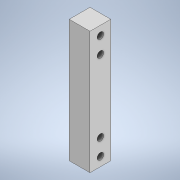
# Autodesk Inventor part: Load_Cell
Saved by Autodesk Inventor 2022 (Build 260153000, 153)
## iProperties
Created: 2022-09-14
Part Number: Load_Cell
Material: Generic
Document SubType Name: Modeling
Designer: tecssupport
Density: 1 g/cm^3
Appearance: Default
Author: tecssupport
Autodesk Inventor part; units mm, degrees
ref_plane "YZ Plane" through (0, 0, 0) normal (1, 0, 0) x (0, 1, 0)
ref_plane "XZ Plane" through (0, 0, 0) normal (0, 1, 0) x (-1, 0, 0)
ref_plane "XY Plane" through (0, 0, 0) normal (0, 0, 1) x (1, 0, 0)
sketch "Sketch2" plane through (0, 0, 0) normal (1, 0, 0) x (0, 1, 0)
  line L0 (37.5, 6.35) -> (-37.5, 6.35)
  line L1 (-37.5, 6.35) -> (-37.5, -6.35)
  line L2 (-37.5, -6.35) -> (37.5, -6.35)
  line L3 (37.5, -6.35) -> (37.5, 6.35)
  point P0 (0, 0)
  point P1 (0, 6.35)
  point P2 (-37.5, 0)
  dimension "d0" = 75
  dimension "d1" = 12.7
  constraints: 8 end point, 2 midpoint, 2 parallel, 1 horizontal, 1 horizontal alignment, 1 perpendicular, 1 vertical alignment
  measures "d0" distance between parallel lines of L1 L3
  measures "d1" distance of L2.end L0.start
extrude "Extrusion1" add sketch "Sketch2" along normal mid plane 12.7
sketch "Sketch3" plane through (6.35, 0, 0) normal (1, 0, 0) x (0, 0, -1)
  circle A0 centre (0, 32) radius 2
  circle A1 centre (0, 22) radius 2
  line L0 (-6.35, 37.5) -> (-6.35, -37.5) projected
  line L1 (-6.35, 0) -> (6.35, 0) construction
  line L2 (6.35, -37.5) -> (6.35, 37.5) projected
  circle A2 centre (0, -32) radius 2
  circle A3 centre (0, -22) radius 2
  point P0 (0, 0)
  dimension "d4" = 22
  dimension "d5" = 10
  dimension "d6" = 4
  constraints: 4 centre point, 2 end point, 2 midpoint, 2 symmetric about line, 2 vertical alignment, 1 equal radius, 2 other
  measures "d4" distance of point (0, 0) A1.centre
  measures "d5" distance of A1.centre A0.centre
  measures "d6" diameter of A1
extrude "Extrusion2" cut sketch "Sketch3" against normal through all
body "Solid1"
